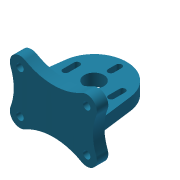
# Autodesk Inventor part: xScrewMount
Saved by Autodesk Inventor 2014 (Build 180170000, 170)
## iProperties
Created: 2014-08-29
Part Number: xScrewMount
Material: Generic
Document SubType Name: Modeling
Designer: Peele
Density: 1 g/cm^3
Appearance: Turquoise
Author: Peele
Autodesk Inventor part; units mm, degrees
ref_plane "YZ Plane" through (0, 0, 0) normal (1, 0, 0) x (0, 1, 0)
ref_plane "XZ Plane" through (0, 0, 0) normal (0, 1, 0) x (-1, 0, 0)
ref_plane "XY Plane" through (0, 0, 0) normal (0, 0, 1) x (1, 0, 0)
sketch "Sketch1" plane through (0, 0, 0) normal (0, 1, 0) x (-1, 0, 0)
  line L0 (-20.5, -13) -> (20.5, -13) construction
  line L1 (20.5, -13) -> (20.5, 13) construction
  line L2 (20.5, 13) -> (-20.5, 13) construction
  line L3 (-20.5, 13) -> (-20.5, -13) construction
  line L4 (-20.5, -13) -> (20.5, 13) construction
  line L5 (20.5, -13) -> (-20.5, 13) construction
  circle A0 centre (-20.5, 13) radius 2.25
  circle A1 centre (20.5, 13) radius 2.25
  circle A2 centre (20.5, -13) radius 2.25
  circle A3 centre (-20.5, -13) radius 2.25
  arc A4 (-26.3343, -10.7586) -> (-26.3343, 10.7586) centre (-54.3388, 0) ccw
  arc A5 (-17.3939, 18.4235) -> (-26.3343, 10.7586) centre (-20.5, 13) ccw
  arc A6 (-17.3939, 18.4235) -> (17.3939, 18.4235) centre (0, 48.7954) ccw
  arc A7 (26.3343, 10.7586) -> (17.3939, 18.4235) centre (20.5, 13) ccw
  arc A8 (-26.3343, -10.7586) -> (-17.3939, -18.4235) centre (-20.5, -13) ccw
  arc A9 (17.3939, -18.4235) -> (-17.3939, -18.4235) centre (0, -48.7954) ccw
  arc A10 (17.3939, -18.4235) -> (26.3343, -10.7586) centre (20.5, -13) ccw
  arc A11 (26.3343, 10.7586) -> (26.3343, -10.7586) centre (54.3388, 0) ccw
  point P0 (0, 0)
  dimension "d0" = 26
  dimension "d1" = 41
  dimension "d2" = 4.5
  dimension "d3" = 4
  dimension "d4" = 30
  dimension "d5" = 35
  constraints: 16 point on circle, 12 centre point, 12 end point, 8 equal radius, 8 tangent, 4 coincident, 4 concentric, 2 midpoint, 2 parallel, 1 horizontal, 1 perpendicular
  measures "d0" distance of L2.end L0.start
  measures "d1" distance of L1.end L2.end
  measures "d2" diameter of A1
  measures "d3" radial gap between concentric circles of A5 A0
  measures "d4" radius of A4
  measures "d5" radius of A9
extrude "Extrusion1" add sketch "Sketch1" along normal blind 7
sketch "Sketch2" plane through (0, 0, 0) normal (0, 0, 1) x (1, 0, 0)
  line L0 (-22.5, 7) -> (22.5, 7)
  line L1 (22.5, 7) -> (19.8341, 27.5704)
  line L2 (-19.8341, 27.5704) -> (-22.5, 7)
  arc A0 (19.8341, 27.5704) -> (-19.8341, 27.5704) centre (0, 25) ccw
  line L3 (-17.3939, 7) -> (17.3939, 7) projected
  point P0 (0, 0)
  dimension "d8" = 20
  dimension "d9" = 18
  dimension "d10" = 45
  constraints: 6 end point, 2 point on circle, 2 tangent, 1 centre point, 1 equal length, 1 horizontal, 1 point on line, 1 vertical alignment
  measures "d8" radius of A0
  measures "d9" distance from line of A0.centre L0
  measures "d10" distance of L0.start L0.end
extrude "Extrusion2" add sketch "Sketch2" along normal mid plane 7.5
sketch "Sketch3" plane through (0, 0, 3.75) normal (0, 0, 1) x (1, 0, 0)
  arc A0 (19.8341, 27.5704) -> (-19.8341, 27.5704) centre (0, 25) ccw projected
  circle A1 centre (0, 25) radius 6
  point P0 (0, 0)
  dimension "d13" = 12
  constraints: 1 centre point, 1 coincident
  measures "d13" diameter of A1
extrude "Extrusion3" cut sketch "Sketch3" against normal through all
sketch "Sketch4" plane through (0, 0, -3.75) normal (0, 0, -1) x (-1, 0, 0)
  circle A0 centre (0, 25) radius 6 projected
  line L0 (22.5, 7) -> (-22.5, 7) projected
  arc A1 (19.8341, 27.5704) -> (-19.8341, 27.5704) centre (0, 25) ccw projected
  line L1 (0, 35.3) -> (0, 40.3) construction
  line L2 (-1.8, 35.3) -> (-1.8, 40.3)
  line L3 (1.8, 40.3) -> (1.8, 35.3)
  arc A2 (-1.8, 35.3) -> (1.8, 35.3) centre (0, 35.3) ccw
  arc A3 (1.8, 40.3) -> (-1.8, 40.3) centre (0, 40.3) ccw
  line L4 (0, 9.7) -> (0, 14.7) construction
  line L5 (-1.8, 9.7) -> (-1.8, 14.7)
  line L6 (1.8, 14.7) -> (1.8, 9.7)
  arc A4 (-1.8, 9.7) -> (1.8, 9.7) centre (0, 9.7) ccw
  arc A5 (1.8, 14.7) -> (-1.8, 14.7) centre (0, 14.7) ccw
  line L7 (-14, 21.5) -> (-14, 28.5) construction
  line L8 (-15.8, 21.5) -> (-15.8, 28.5)
  line L9 (-12.2, 28.5) -> (-12.2, 21.5)
  arc A6 (-15.8, 21.5) -> (-12.2, 21.5) centre (-14, 21.5) ccw
  arc A7 (-12.2, 28.5) -> (-15.8, 28.5) centre (-14, 28.5) ccw
  line L10 (14, 21.5) -> (14, 28.5) construction
  line L11 (12.2, 21.5) -> (12.2, 28.5)
  line L12 (15.8, 28.5) -> (15.8, 21.5)
  arc A8 (12.2, 21.5) -> (15.8, 21.5) centre (14, 21.5) ccw
  arc A9 (15.8, 28.5) -> (12.2, 28.5) centre (14, 28.5) ccw
  point P0 (0, 0)
  point P1 (0, 37.8)
  point P2 (0, 12.2)
  point P3 (-14, 25)
  point P4 (14, 25)
  dimension "d16" = 3.6
  dimension "d17" = 5
  dimension "d18" = 2.5
  dimension "d19" = 2.5
  dimension "d20" = 14
  dimension "d21" = 14
  dimension "d22" = 7
  constraints: 32 end point, 16 point on circle, 16 tangent, 8 centre point, 6 parallel, 4 midpoint, 3 equal radius, 2 equal length, 2 horizontal alignment, 2 vertical alignment, 1 collinear, 1 perpendicular
  measures "d16" distance between parallel lines of L2 L3
  measures "d17" distance of L1.start L1.end
  measures "d20" distance from line of A0.centre L7
  measures "d21" distance from line of L10 A1.centre
  measures "d22" distance of L8.start L8.end
extrude "Extrusion4" cut sketch "Sketch4" against normal blind 7.5 contours L2 A3 L3 A2 | L5 A5 L6 A4 | L8 A7 L9 A6 | L11 A9 L12 A8
equation "\"d19\" = d18"
equation "\"d21\" = d20"
body "Solid1"
